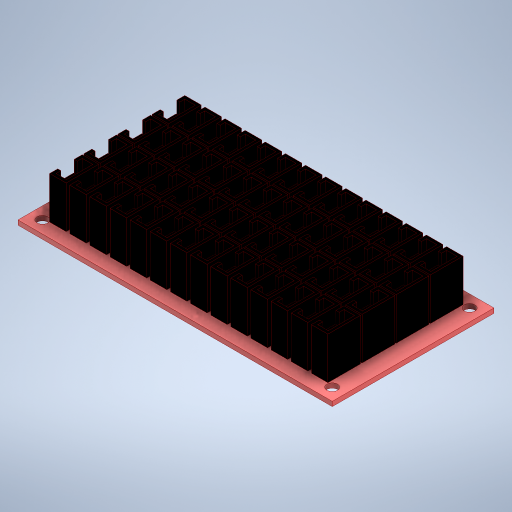
# Autodesk Inventor part: Conector IC DC
Saved by Autodesk Inventor 2024.2 (Build 282272000, 272)
## iProperties
Created: 2024-08-27
Part Number: Conector IC DC
Material: Phenolic Resin
Document SubType Name: Modeling
Designer: ja.restrepo1
Density: 1.38 g/cm^3
Appearance: Smooth - Red
Author: ja.restrepo1
Autodesk Inventor part; units mm, degrees
ref_plane "YZ Plane" through (0, 0, 0) normal (1, 0, 0) x (0, 1, 0)
sketch "Sketch1" plane through (0, 0, 0) normal (0, 1, 0) x (-1, 0, 0)
  line L0 (51.5, -26.5) -> (-51.5, -26.5)
  line L1 (-51.5, -26.5) -> (-51.5, 26.5)
  line L2 (-51.5, 26.5) -> (51.5, 26.5)
  line L3 (51.5, 26.5) -> (51.5, -26.5)
  circle A0 centre (47.5, -22.5) radius 1.75
  circle A1 centre (-47.5, -22.5) radius 1.75
  circle A2 centre (-47.5, 22.5) radius 1.75
  circle A3 centre (47.5, 22.5) radius 1.75
  line L4 (47.5, -22.5) -> (-47.5, -22.5) construction
  line L5 (-47.5, -22.5) -> (-47.5, 22.5) construction
  point P0 (0, 0)
  point P1 (-51.5, 0)
  point P2 (0, -26.5)
  point P3 (-47.5, 0)
  point P4 (0, -22.5)
  dimension "d0" = 103
  dimension "d1" = 53
  dimension "d2" = 3.5
  dimension "d3" = 95
  dimension "d4" = 45
  constraints: 12 end point, 4 centre point, 4 horizontal alignment, 4 midpoint, 4 vertical alignment, 3 equal radius, 2 horizontal, 2 parallel, 2 perpendicular
  measures "d0" distance of L1.end L2.end
  measures "d1" distance of L0.end L1.end
  measures "d2" diameter of A0
  measures "d3" distance of L4.start L4.end
  measures "d4" distance of L4.end L5.end
extrude "Extrusion1" add sketch "Sketch1" along normal mid plane 1.5
ref_plane "Work Plane1" through (0, 14.75, 0) normal (0, 1, 0) x (1, 0, 0)
sketch "Sketch3" plane through (0, 14.75, 0) normal (0, 1, 0) x (1, 0, 0)
  line L0 (-45.49, -11.45) -> (-40.09, -11.45)
  line L1 (-40.09, -11.45) -> (-40.09, -22.15)
  line L2 (-40.09, -22.15) -> (-45.49, -22.15)
  line L3 (-45.49, -22.15) -> (-45.49, -19.5)
  line L4 (-45.49, -14.1) -> (-44.43, -14.1)
  line L5 (-44.43, -14.1) -> (-44.43, -12.5)
  line L6 (-44.43, -12.5) -> (-41, -12.5)
  line L7 (-41, -12.5) -> (-41, -21.1)
  line L8 (-41, -21.1) -> (-44.43, -21.1)
  line L9 (-44.43, -21.1) -> (-44.43, -19.5)
  line L10 (-44.43, -19.5) -> (-45.49, -19.5)
  line L11 (-45.49, -14.1) -> (-45.49, -11.45)
  line L12 (-45.49, -19.5) -> (-45.49, -14.1)
  line L13 (-45.49, -14.1) -> (-45.69, -14.1)
  line L14 (-45.69, -14.1) -> (-45.69, -19.5)
  line L15 (-45.69, -19.5) -> (-45.49, -19.5)
  point P0 (0, 0)
  point P1 (-41, -16.8)
  dimension "d14" = 5.4
  dimension "d15" = 10.7
  dimension "d16" = 5.4
  dimension "d17" = 1.06
  dimension "d18" = 3.43
  dimension "d19" = 8.6
  dimension "d20" = 41
  dimension "d21" = 16.8
  dimension "d28" = 5.35
  dimension "d31" = 0.2
  constraints: 32 end point, 10 perpendicular, 4 parallel, 3 horizontal, 2 point on line, 1 collinear, 1 midpoint
  measures "d14" distance of L1.end L2.end
  measures "d15" distance of L0.end L1.end
  measures "d16" distance between parallel lines of L10 L4
  measures "d17" distance of L4.start L4.end
  measures "d18" distance of L5.end L6.end
  measures "d19" distance of L6.end L7.end
  measures "d20" horizontal distance of point (0, 0) point (-41, -16.8)
  measures "d21" vertical distance of point (0, 0) point (-41, -16.8)
  measures "d28" distance from line of L0 point (-41, -16.8)
  measures "d31" distance between parallel lines of L14 L12
extrude "Sock connector" add sketch "Sketch3" against normal blind 13.8 separate body
sketch "Sketch4" plane through (0, 14.75, 0) normal (0, 1, 0) x (1, 0, 0)
  line L0 (-45.49, -14.1) -> (-44.43, -14.1)
  line L1 (-44.43, -14.1) -> (-44.43, -12.5)
  line L2 (-44.43, -12.5) -> (-41, -12.5)
  line L3 (-41, -12.5) -> (-41, -21.1)
  line L4 (-41, -21.1) -> (-44.43, -21.1)
  line L5 (-44.43, -21.1) -> (-44.43, -19.5)
  line L6 (-44.43, -19.5) -> (-45.49, -19.5)
  line L7 (-45.49, -19.5) -> (-45.49, -14.1)
  line L8 (-45.49, -14.1) -> (-45.69, -14.1)
  line L9 (-45.69, -14.1) -> (-45.69, -19.5)
  line L10 (-45.69, -19.5) -> (-45.49, -19.5)
  line L11 (-45.49, -19.5) -> (-45.49, -22.15) projected
  line L12 (-40.09, -22.15) -> (-40.09, -11.45) projected
  point P0 (0, 0)
  point P1 (-41, -16.8)
  point P2 (-40.09, -16.8)
  dimension "d38" = 5.4
  dimension "d39" = 1.06
  dimension "d40" = 3.43
  dimension "d41" = 8.6
  dimension "d42" = 0.2
  constraints: 22 end point, 7 perpendicular, 2 collinear, 2 horizontal, 2 midpoint, 2 point on line, 1 horizontal alignment
  measures "d38" distance between parallel lines of L6 L0
  measures "d39" distance of L8.start L0.end
  measures "d40" distance of L1.end L2.end
  measures "d41" distance of L2.end L4.start
  measures "d42" distance between parallel lines of L9 L7
extrude "connector" cut sketch "Sketch4" against normal blind 4 bodies 2
pattern_linear "Rectangular Pattern1" count 14 spacing 6.6 along (1, 0, 0) count 4 spacing 11.2 along (0, 0, -1) of "Sock connector", "connector" bodies 2
ref_plane "Work Plane2" through (0, -8.75, 0) normal (0, -1, 0) x (1, 0, 0)
sketch "Sketch7" plane through (0, -8.75, 0) normal (0, -1, 0) x (1, 0, 0)
  line L0 (-32.9, 2.75) -> (30.9, 2.75)
  line L1 (30.9, 2.75) -> (30.9, -2.75)
  line L2 (30.9, -2.75) -> (-32.9, -2.75)
  line L3 (-32.9, -2.75) -> (-32.9, 2.75)
  line L4 (-31.25, 0.8) -> (29.25, 0.8)
  line L5 (29.25, 0.8) -> (29.25, -0.8)
  line L6 (29.25, -0.8) -> (-31.25, -0.8)
  line L7 (-31.25, -0.8) -> (-31.25, 0.8)
  point P0 (0, 0)
  point P1 (-1, 0.8)
  point P2 (-1, 2.75)
  point P3 (29.25, 0)
  point P4 (30.9, 0)
  dimension "d52" = 63.8
  dimension "d53" = 5.5
  dimension "d54" = 60.5
  dimension "d55" = 1.6
  dimension "d62" = 1
  constraints: 16 end point, 4 midpoint, 4 parallel, 2 horizontal alignment, 2 perpendicular, 2 vertical, 1 vertical alignment
  measures "d52" distance of L1.end L2.end
  measures "d53" distance of L0.end L1.end
  measures "d54" distance of L5.end L6.end
  measures "d55" distance of L4.end L5.end
  measures "d62" horizontal distance of point (-1, 0.8) point (0, 0)
extrude "Conector tarjeta" add sketch "Sketch7" against normal blind 8 separate body contours L0 L1 L2 L3 | L4 L5 L6 L7
extrude "ranura conector" add sketch "Sketch7" against normal blind 6.5 contours L4 L5 L6 L7 bodies 1
